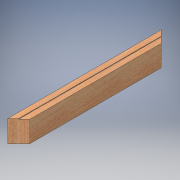
# Autodesk Inventor part: SideWidth
Saved by Autodesk Inventor 2016 (Build 200138000, 138)
## iProperties
Created: 2016-02-09
Part Number: SideWidth
Material: Wood (Birch)
Document SubType Name: Modeling
Designer: ron
Density: 0.55 g/cm^3
Appearance: Birch - Natural Polished
Author: ron
Autodesk Inventor part; units mm, degrees
ref_plane "YZ Plane" through (0, 0, 0) normal (1, 0, 0) x (0, 1, 0)
ref_plane "XZ Plane" through (0, 0, 0) normal (0, 1, 0) x (-1, 0, 0)
ref_plane "XY Plane" through (0, 0, 0) normal (0, 0, 1) x (1, 0, 0)
sketch "Sketch1" plane through (0, 0, 0) normal (0, 0, 1) x (1, 0, 0)
  line L0 (0, 0) -> (0, 101.6)
  line L1 (0, 101.6) -> (25.4, 101.6)
  line L2 (25.4, 101.6) -> (25.4, 98.6028)
  line L3 (25.4, 98.6028) -> (50.8, 98.6028)
  line L4 (50.8, 98.6028) -> (50.8, 0)
  line L5 (50.8, 0) -> (0, 0)
  dimension "d0" = 101.6
  dimension "d1" = 25.4
  dimension "d2" = 2.9972
  dimension "d3" = 25.4
  constraints: 12 end point, 5 perpendicular, 1 vertical
  measures "d0" distance of L0.start L0.end
  measures "d1" distance of L0.end L1.end
  measures "d2" distance of L1.end L2.end
  measures "d3" distance of L2.end L3.end
extrude "Extrusion1" add sketch "Sketch1" along normal blind 711.2
chamfer "Chamfer1" distance 50.8 angle 45 1 edges at (50.8, 49.3014, 711.2)
chamfer "Chamfer2" distance 50.8 angle 45 1 edges at (50.8, 49.3014, 0)
body "Solid1"
